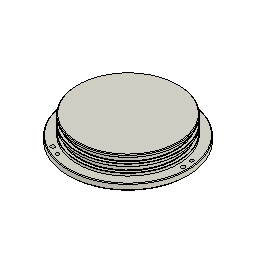
end_cap_blank (Autodesk Fusion 360 design; units mm, degrees)
Autodesk Fusion 360 part; units mm, degrees
sketch "Sketch1" plane through (0, 0, 0) normal (0, 1, 0) x (1, 0, 0)
  line L0 (0, 0) -> (45, 0)
  line L1 (45, 0) -> (45, -5)
  line L2 (45, -5) -> (38, -5)
  line L3 (38, -19) -> (0, -19)
  line L4 (0, -19) -> (0, 0)
  line L5 (38, -7) -> (35.7, -7)
  line L6 (35.7, -7) -> (35.7, -11)
  line L7 (35.7, -11) -> (38, -11)
  line L8 (38, -13) -> (35.7, -13)
  line L9 (35.7, -13) -> (35.7, -17)
  line L10 (35.7, -17) -> (38, -17)
  line L11 (38, -5) -> (38, -7)
  line L12 (38, -11) -> (38, -13)
  line L13 (38, -17) -> (38, -19)
  dimension "d2" = 45
  dimension "d4" = 5
  dimension "d5" = 7
  dimension "d9" = 4
  dimension "d10" = 4
  dimension "d11" = 2.3
  dimension "d13" = 2
  dimension "d14" = 2
  dimension "d15" = 2
  dimension "d16" = 19
  constraint coincident L0.start L4.end
  constraint horizontal L0
  constraint perpendicular L0 L1
  constraint perpendicular L1 L2
  constraint perpendicular L2 L11
  constraint perpendicular L1 L3
  constraint perpendicular L0 L4
  constraint perpendicular L5 L11
  constraint perpendicular L5 L6
  constraint perpendicular L7 L11
  constraint coincident L8.start L11
  constraint perpendicular L8 L11
  constraint perpendicular L8 L9
  constraint coincident L10.end L11
  constraint perpendicular L10 L11
  constraint collinear L11 L12
  constraint coincident L7.end L11
  constraint collinear L6 L9
  constraint collinear L12 L13
  measures "d2" distance of L0.start L0.end
  measures "d4" distance of L0.end L1.end
  measures "d5" distance of L1.end L2.end
  measures "d9" distance of L5.end L6.end
  measures "d10" distance of L8.end L9.end
  measures "d11" distance of L8.start L8.end
  measures "d13" distance of L3.start L10.end
  measures "d14" distance of L7.end L8.start
  measures "d15" distance of L2.end L5.start
  measures "d16" distance of L3.end L0.start
revolve "Revolve1" add sketch "Sketch1" angle 360 about axis through (0, 0, 19) along (0, 0, -1)
chamfer "Chamfer1" distance 1 angle 45 1 edges at (-41.9547, -16.2727, 0)
chamfer "Chamfer2" distance 0.5 angle 45 1 edges at (-35.4284, -13.7414, 19)
fillet "Fillet1" radius 0.2 4 edges at (-35.4284, -13.7414, 17) (-35.4284, -13.7414, 13) (-35.4284, -13.7414, 11) (-35.4284, -13.7414, 7)
fillet "Fillet2" radius 0.3 2 faces at (35.6556, 1.7795, 14.3333) (35.6556, 1.7795, 9.6667)
sketch "Sketch3" plane through (0, 0, 0) normal (0, 0, -1) x (1, 0, 0)
  circle A0 centre (0, 0) radius 44
  point P0 (41.5, 0)
  point P1 (40.8695, -7.2064)
  dimension "d50" = 41.5
  dimension "d51" = 41.5
  dimension "d52" = 10
  constraint horizontal A0.centre P0
  measures "d50" distance of A0.centre P0
  measures "d51" distance of A0.centre P1
  measures "d52" angle of A0.centre P0 P1
hole "Hole4" at (40.8695, 7.2064, 0) direction (0, 0, 1) diameter 2.529 end through all
thread "Thread3" "ISO Metric profile 3.0 M3x0.5 6H" thread offset 0 thread depth 10
hole "Hole5" at (41.5, 0, 0) direction (0, 0, 1) diameter 3 end through all
pattern_circular "C-Pattern6" count 3 over 360 about axis through (0, 0, 1.75) along (0, 0, 1) of "Hole4", "Hole5"
chamfer "Chamfer3" distance 0.5 angle 45 1 edges at (-41.9547, -16.2727, 5)
equation "D_i = 76 mm" comment "Inner Diameter of Cylinder"
equation "d2 = ( D_i + 2 * t ) / 2"
equation "t = 7 mm" comment "Thickness of cylinder wall"
equation "d5 = t"
equation "Oring_depth = 2.3 mm" comment "Depth of Oring Groove"
equation "Oring_width = 4 mm" comment "Width of Oring Groove"
equation "d9 = Oring_width"
equation "d10 = Oring_width"
equation "d11 = Oring_depth"
equation "d50 = D_i / 2 + t / 2"
equation "d51 = d50"
